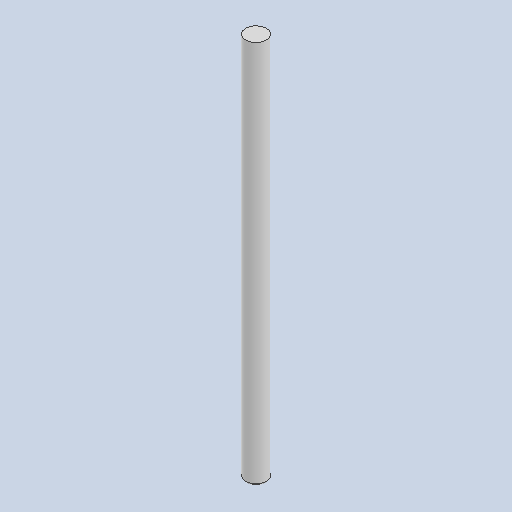
# Autodesk Inventor part: Rotor
Saved by Autodesk Inventor 2022.2 (Build 262287000, 287)
## iProperties
Created: 2021-01-20
Part Number: Rotor
Material: Genérico
Document SubType Name: Modeling
Designer: João
Density: 1 g/cm^3
Appearance: Padrão
Mass: 0.014602 g
Surface Area: 0.598651 cm^2
Volume: 0.014602 cm^3
Author: João
Autodesk Inventor part; units mm, degrees
ref_plane "YZ Plane" through (0, 0, 0) normal (1, 0, 0) x (0, 1, 0)
ref_plane "XZ Plane" through (0, 0, 0) normal (0, 1, 0) x (-1, 0, 0)
ref_plane "XY Plane" through (0, 0, 0) normal (0, 0, 1) x (1, 0, 0)
sketch "Esboço1" plane through (0, 0, 0) normal (0, 1, 0) x (-1, 0, 0)
  circle A0 centre (0, 0) radius 0.5
  dimension "d0" = 1
  constraints: 1 centre point, 1 coincident
  measures "d0" diameter of A0
extrude "Extrusão1" add sketch "Esboço1" along normal blind 18.6
fillet "Arredondamento2" radius 0.1 1 edges at (0.5, 0, 0)
